Autodesk Fusion 360 part; units mm, degrees
(part 2 of 2)
sketch "Sketch8" plane through (1219.2, 0, 0) normal (1, 0, 0) x (0, 1, 0)
  line L0 (80.01, 0) -> (0, 0)
  line L1 (0, 0) -> (0, -203.2)
  line L2 (0, -203.2) -> (73.66, -203.2)
  line L3 (73.66, -203.2) -> (80.01, -196.85)
  line L4 (80.01, -196.85) -> (80.01, 0)
  line L5 (80.01, 0) -> (80.01, -6.35)
  line L6 (80.01, 0) -> (73.66, 0)
  line L7 (80.01, -6.35) -> (73.66, 0)
  dimension "d49" = 6.35
  dimension "d50" = 6.35
  constraint coincident L0.start L4.end
  constraint perpendicular L0 L5
  constraint perpendicular L5 L6
  measures "d49" distance of L0.start L5.end
  measures "d50" distance of L0.start L6.end
extrude "Extrude8" cut sketch "Sketch8" against normal blind 2438.4 contours L0 L4 L5 L6 L7 bodies 6
fillet "Fillet4" radius 2.54 1 edges at (0, 45.72, -41.91) on bodies 6
split "Split5" by plane through (1216.025, 0, 0) normal (-1, 0, 0) bodies 6 makes body 9 at (402.8732, 3.175, -67.7333)
split "Split6" by plane through (-1216.025, 0, 0) normal (1, 0, 0) bodies 9 makes body 10 at (402.8732, 3.175, -67.7333)
fillet "Fillet5" radius 2.54 8 edges at (0, 45.72, 0) (1214.9943, -1.1751, 0) (1214.12, 0, 0) (1211.7483, 2.3508, 0) (0, 3.175, 0) (-1211.7483, 2.3508, 0) (-1214.12, 0, 0) (-1214.9943, -1.1751, 0) on bodies 10
fillet "Fillet6" radius 2.54 13 edges at (-1214.9978, -1.1787, -101.748) (-1214.1199, 0.0001, -101.6738) (-1213.5803, 0.7892, -101.6269) (-1210.9886, 2.7166, -101.6) (0, 3.175, -101.6) (1210.9886, 2.7166, -101.6) (1213.5803, 0.7892, -101.6269) (1214.1199, 0.0001, -101.6738) (1214.9978, -1.1787, -101.748) (-1215.0951, 71.12, -102.5299) (0, 71.12, -101.6) (1215.0951, 71.12, -102.5299) (0, 71.12, -41.91) on bodies 10
fillet "Fillet7" radius 1.5875 42 edges at (1235.2852, -3.175, 0) (1217.7381, -2.8896, 0) (1254.125, -3.175, -3.175) (1257.3, -3.175, -101.6) (1257.3, 0, -101.6) (1254.125, 0, -3.175) (1235.075, 0, 0) (1219.2, 36.83, 0) (1254.125, 0, -200.025) (1254.125, -3.175, -200.025) (1219.2, 36.83, -203.2) (1235.075, 0, -203.2) (1216.025, 38.4175, -203.2) (1217.8849, -1.3151, -203.2) (1236.6625, -3.175, -203.2) (1216.025, 76.835, -200.025) (1219.2, 76.835, -200.025) (1219.2, 80.01, -101.6) (1216.025, 80.01, -101.6) (1216.025, 76.835, -3.175) (1219.2, 76.835, -3.175) (-1235.2852, -3.175, 0) (-1217.7381, -2.8896, 0) (-1254.125, -3.175, -3.175) (-1257.3, -3.175, -101.6) (-1254.125, -3.175, -200.025) (-1216.025, 38.4175, -203.2) (-1217.8849, -1.3151, -203.2) (-1236.6625, -3.175, -203.2) (-1216.025, 76.835, -200.025) (-1216.025, 80.01, -101.6) (-1216.025, 76.835, -3.175) (-1219.2, 36.83, 0) (-1235.075, 0, 0) (-1254.125, 0, -3.175) (-1257.3, 0, -101.6) (-1254.125, 0, -200.025) (-1235.075, 0, -203.2) (-1219.2, 36.83, -203.2) (-1219.2, 76.835, -200.025) (-1219.2, 80.01, -101.6) (-1219.2, 76.835, -3.175) on bodies 6 9
combine "Combine2" operation add target body 10 tool bodies 9 6
sketch "Sketch9" plane through (0, -3.175, 0) normal (0, -1, 0) x (1, 0, 0)
  line L0 (1250.2924, -1.5875) -> (1219.6203, -1.5875)
  line L1 (1219.6203, -1.5875) -> (1219.6203, -102.9574)
  spline S0 degree 3 poles (1222.375, -104.775) (1221.7455, -104.3299) (1221.0537, -103.839) (1220.1014, -103.2396) (1219.8611, -103.0952) (1219.6203, -102.9574) knots 0 0 0 0 0.231281 0.231281 0.308124 0.308124 0.308124 0.308124
  line L2 (1222.375, -104.775) -> (1222.375, -201.6125)
  line L3 (1222.375, -201.6125) -> (1250.2924, -201.6125)
  line L4 (1250.2924, -201.6125) -> (1255.7125, -196.1924)
  line L5 (1255.7125, -196.1924) -> (1255.7125, -7.0076)
  line L6 (1255.7125, -7.0076) -> (1250.2924, -1.5875)
  arc A0 (1217.7886, -0.0098) -> (1217.6125, 0) centre (1217.6125, -1.5875) ccw
  spline S1 degree 3 poles (1222.375, -203.2) (1222.329, -203.2) (1222.2831, -203.2) (1222.1838, -203.2) (1222.1305, -203.2) (1221.8497, -203.2) (1221.6226, -203.1999) (1221.1455, -203.1984) (1220.8962, -203.1967) (1220.2906, -203.1858) (1219.937, -203.1738) (1219.2149, -203.1178) (1218.844, -203.0711) (1218.4712, -202.9837) (1218.4503, -202.9787) (1218.4296, -202.9736) knots -0.428714 -0.428714 -0.428714 -0.428714 -0.420839 -0.420839 -0.411701 -0.411701 -0.372681 -0.372681 -0.32947 -0.32947 -0.267016 -0.267016 -0.199248 -0.199248 -0.195185 -0.195185 -0.195185 -0.195185
  spline S2 degree 3 poles (1217.7886, -0.0098) (1218.3472, 0.0022) (1218.9533, 0) (1219.6077, 0) (1219.614, 0) (1219.6203, 0) knots -0.194415 -0.194415 -0.194415 -0.194415 0 0 0.001894 0.001894 0.001894 0.001894
  arc A1 (1216.025, -201.6125) -> (1218.4296, -202.9736) centre (1217.6125, -201.6125) ccw
  line L7 (1216.025, -201.6125) -> (1216.025, -196.1924)
  line L8 (1216.025, -196.1924) -> (1216.025, -104.775)
  line L9 (1216.025, 0) -> (1217.6125, 0)
  line L10 (-1216.025, -196.1924) -> (-1216.025, -201.6125)
  line L11 (-1216.025, -104.775) -> (-1216.025, -196.1924)
  arc A2 (-1217.6125, 0) -> (-1217.7886, -0.0098) centre (-1217.6125, -1.5875) ccw
  spline S3 degree 3 poles (-1219.6203, 0) (-1219.614, 0) (-1219.6077, 0) (-1218.9533, 0) (-1218.3471, 0.0022) (-1217.7886, -0.0098) knots -0.311751 -0.311751 -0.311751 -0.311751 -0.310364 -0.310364 -0.167936 -0.167936 -0.167936 -0.167936
  arc A3 (-1218.4296, -202.9736) -> (-1216.025, -201.6125) centre (-1217.6125, -201.6125) ccw
  spline S4 degree 3 poles (-1218.4296, -202.9736) (-1218.4503, -202.9787) (-1218.4712, -202.9837) (-1218.844, -203.0711) (-1219.2149, -203.1178) (-1219.937, -203.1738) (-1220.2906, -203.1858) (-1220.8962, -203.1967) (-1221.1455, -203.1984) (-1221.6226, -203.1999) (-1221.8497, -203.2) (-1222.1305, -203.2) (-1222.1838, -203.2) (-1222.2831, -203.2) (-1222.329, -203.2) (-1222.375, -203.2) knots -0.395015 -0.395015 -0.395015 -0.395015 -0.387901 -0.387901 -0.269271 -0.269271 -0.159944 -0.159944 -0.084301 -0.084301 -0.015995 -0.015995 0 0 0.013786 0.013786 0.013786 0.013786
  line L12 (-1217.6125, 0) -> (-1216.025, 0)
  arc A4 (1216.025, -104.775) -> (1212.85, -101.6) centre (1212.85, -104.775) ccw
  line L13 (1212.85, -101.6) -> (-1212.85, -101.6)
  arc A5 (-1212.85, -101.6) -> (-1216.025, -104.775) centre (-1212.85, -104.775) ccw
  line L14 (-1216.025, 0) -> (1216.025, 0)
  line L15 (1250.95, 0) -> (1219.6203, 0)
  line L16 (1257.3, -6.35) -> (1250.95, 0)
  line L17 (1257.3, -196.85) -> (1257.3, -6.35)
  line L18 (1250.95, -203.2) -> (1257.3, -196.85)
  line L19 (1222.375, -203.2) -> (1250.95, -203.2)
  line L20 (-1222.375, -203.2) -> (-1250.95, -203.2)
  line L21 (-1250.95, -203.2) -> (-1257.3, -196.85)
  line L22 (-1257.3, -196.85) -> (-1257.3, -6.35)
  line L23 (-1250.95, 0) -> (-1219.6203, 0)
  line L24 (-1257.3, -6.35) -> (-1250.95, 0)
equation "d3 = 1 5/8\""
equation "d60 = ( 1 / 16 ) * 1 in"
